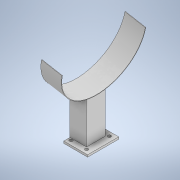
# Autodesk Inventor part: 零件1
Saved by Autodesk Inventor 2020 (Build 240168000, 168)
## iProperties
Created: 2020-11-23
Part Number: 零件1
Material: 常规
Document SubType Name: Sheet Metal
Designer: huang
Density: 1 g/cm^3
Sheet Metal Rule: 默认_mm
Appearance: 默认
Author: huang
## iProperties of the stored document _3D 打印.ipt
Created: 2020-11-23
Part Number: _3D 打印
Material: 常规
Document SubType Name: Modeling
Designer: huang
Density: 1 g/cm^3
Appearance: 默认
Author: huang
Autodesk Inventor part; units mm, degrees
ref_plane "YZ Plane" through (0, 0, 0) normal (1, 0, 0) x (0, 1, 0)
ref_plane "XZ Plane" through (0, 0, 0) normal (0, 1, 0) x (-1, 0, 0)
sketch "草图1" plane through (0, 0, 0) normal (0, 1, 0) x (-1, 0, 0)
  line L0 (20.0444, 13.4444) -> (-9.9556, 13.4444)
  line L1 (-9.9556, 13.4444) -> (-9.9556, -16.5556)
  line L2 (-9.9556, -16.5556) -> (20.0444, -16.5556)
  line L3 (20.0444, -16.5556) -> (20.0444, 13.4444)
  line L4 (0.0444, 13.4444) -> (-7.4556, 13.4444)
  line L5 (0.0444, 13.4444) -> (7.5444, 13.4444)
  dimension "d0" = 30
  dimension "d1" = 30
  constraints: 12 end point, 3 point on line, 2 parallel, 1 horizontal, 1 perpendicular
  measures "d0" distance of L0.start L0.end
  measures "d1" distance of L0.end L1.end
extrude "拉伸1" add sketch "草图1" along normal blind 2
sketch "草图2" plane through (0, 2, 0) normal (0, 1, 0) x (1, 0, 0)
  line L0 (9.9556, 16.5556) -> (-20.0444, 16.5556) projected
  circle A0 centre (4.9556, 12.5556) radius 1.5
  circle A1 centre (-10.0444, 12.5556) radius 1.5
  circle A2 centre (-10.0444, -9.4444) radius 1.5
  circle A3 centre (4.9556, -9.4444) radius 1.5
  line L1 (-10.0444, 12.5556) -> (-10.0444, 16.5556)
  line L2 (4.9556, 12.5556) -> (4.9556, 16.5556)
  line L3 (-10.0444, -9.4444) -> (-10.0444, -13.4444)
  line L4 (-20.0444, -13.4444) -> (9.9556, -13.4444) projected
  line L5 (4.9556, -9.4444) -> (4.9556, -13.4444)
  line L6 (9.9556, -13.4444) -> (9.9556, 16.5556) projected
  line L7 (-20.0444, 16.5556) -> (-20.0444, -13.4444) projected
  point P0 (0, 0)
  dimension "d15" = 3
  dimension "d16" = 3
  dimension "d17" = 3
  dimension "d108" = 4
  dimension "d109" = 4
  dimension "d110" = 4
  dimension "d111" = 4
  dimension "d112" = 5
  dimension "d113" = 10
  constraints: 8 end point, 6 point on line, 4 centre point, 2 perpendicular
  measures "d15" diameter of A0
  measures "d16" diameter of A1
  measures "d17" diameter of A2
  measures "d108" distance of L1.start L1.end
  measures "d109" distance of L2.start L2.end
  measures "d110" distance of L5.start L5.end
  measures "d111" distance of L3.start L3.end
  measures "d112" distance from line of L6 L2.start
  measures "d113" distance from line of L7 L1.start
extrude "拉伸2" cut sketch "草图2" against normal blind 2 contours A0 | A1 | A2 | A3
sketch "草图3" plane through (0, 2, 0) normal (0, 1, 0) x (1, 0, 0)
  circle A0 centre (4.9556, 12.5556) radius 1.5 projected
  circle A1 centre (-10.0444, -9.4444) radius 1.5 projected
  line L0 (2.9556, 10.5556) -> (2.9556, -7.4444)
  line L1 (-13.0444, 10.5556) -> (-13.0444, -7.4444)
  line L2 (-13.0444, -7.4444) -> (2.9556, -7.4444)
  line L3 (-13.0444, 10.5556) -> (2.9556, 10.5556)
  line L4 (-22.598, 1.5556) -> (13.9828, 1.5556)
  point P0 (0, 0)
  dimension "d137" = 11
  constraints: 10 end point, 2 horizontal, 1 parallel
  measures "d137" distance from line of A0.centre L4
extrude "拉伸3" add sketch "草图3" along normal blind 60 contours L0 L4 L1 L3 | L0 L2 L1 L4
chamfer "倒角5" distance 16 angle 10 1 edges at (2.9556, 62, -1.5556) measured on face at (-2.3778, 62, 1.4444)
sketch "草图29" plane through (0, 2, 0) normal (0, 1, 0) x (1, 0, 0)
  line L0 (-13.0444, -7.4444) -> (-13.0444, 10.5556) projected
  line L1 (-13.0444, 10.5556) -> (-20.9964, 10.5556)
  line L2 (-20.9964, 10.5556) -> (-20.9964, -16.1821)
  line L3 (-20.9964, -16.1821) -> (-13.0444, -16.1821)
  line L4 (-13.0444, -16.1821) -> (-13.0444, 10.5556)
  line L5 (-13.0444, 10.5556) -> (-22.8537, 10.5556)
  line L6 (-22.8537, 10.5556) -> (-22.8537, 28.4787)
  line L7 (-22.8537, 28.4787) -> (-13.0444, 28.4787)
  line L8 (-13.0444, 28.4787) -> (-13.0444, 10.5556)
  point P0 (0, 0)
  point P1 (-20.0444, -13.4444)
  constraints: 16 end point, 4 parallel, 2 horizontal, 2 perpendicular
extrude "拉伸15" cut sketch "草图29" against normal blind 20
sketch "草图31" plane through (-13.0444, 62, 7.4444) normal (0.1736, 0.9848, 0) x (0.9848, -0.1736, 0)
  line L0 (0, 18) -> (0, 0) projected
  line L1 (0, 9) -> (16.2468, 9)
  line L2 (16.2468, 0) -> (16.2468, 18) projected
  circle A0 centre (8.1234, 9) radius 1.5
  point P0 (23.6125, 7.4444)
  dimension "d134" = 3
  constraints: 3 midpoint, 2 end point, 1 centre point
  measures "d134" diameter of A0
extrude "拉伸16" cut sketch "草图31" against normal blind 20
ref_plane "工作平面4" through (-13.0444, 62, -10.5556) normal (-0.9848, 0.1736, 0) x (0, 0, 1)
ref_plane "工作平面3" through (2.9556, 59.1788, -1.5556) normal (0.1736, 0.9848, 0) x (0.9848, -0.1736, 0)
sketch "草图36" plane through (-13.0444, 62, -10.5556) normal (-0.9848, 0.1736, 0) x (0, 0, 1)
  line L0 (18, 0) -> (0, 0) projected
  circle A0 centre (9, 0) radius 15
  point P0 (10.5556, -58.7929)
  dimension "d140" = 30
  constraints: 1 centre point, 1 midpoint
  measures "d140" diameter of A0
extrude "拉伸17" cut sketch "草图36" against normal blind 200
sketch "草图38" plane through (-13.0444, 62, -10.5556) normal (-0.9848, 0.1736, 0) x (0, 0, 1)
  line L0 (9, -17.5895) -> (9, 63.4105)
  circle A0 centre (9, 22.9105) radius 40.5
  point P0 (10.5556, -58.7929)
  dimension "d143" = 81
  constraints: 2 end point, 1 midpoint, 1 vertical, 1 vertical alignment, 2 other
  measures "d143" distance of L0.start L0.end
extrude "拉伸18" add sketch "草图38" against normal blind 20
sketch "草图39" plane through (-9.0661, 84.5624, -1.5556) normal (-0.9848, 0.1736, 0) x (0, 0, 1)
  line L0 (-48.0605, 0) -> (68.7188, 0)
  line L1 (68.7188, 0) -> (68.7188, 57.1611)
  line L2 (68.7188, 57.1611) -> (-48.0605, 57.1611)
  line L3 (-48.0605, 57.1611) -> (-48.0605, 0)
  point P0 (1.5556, -81.7034)
  constraints: 8 end point, 2 parallel, 1 horizontal, 1 perpendicular
extrude "拉伸19" cut sketch "草图39" against normal through all
sketch "草图41" plane through (-13.0444, 62, -10.5556) normal (-0.9848, 0.1736, 0) x (0, 0, 1)
  line L0 (49.5, 22.9105) -> (-31.5, 22.9105) projected
  circle A0 centre (9, 22.9105) radius 40
  point P0 (10.5556, -58.7929)
  dimension "d148" = 80
  constraints: 1 centre point, 1 midpoint
  measures "d148" diameter of A0
extrude "拉伸20" cut sketch "草图41" against normal blind 20
equation "\"折弯半径\" = 厚度"
equation "\"折弯释压宽度\" = 厚度"
equation "\"折弯释压深度\" = 0.5 * 厚度"
equation "\"拐角释压尺寸\" = 4 * 厚度"
equation "\"最小余量\" = 2 * 厚度"
equation "\"过渡半径\" = 折弯半径"
equation "\"Jacobi半径尺寸\" = 折弯半径"
equation "\"间隙大小\" = 厚度"
equation "\"厚度\" = 0.5"
